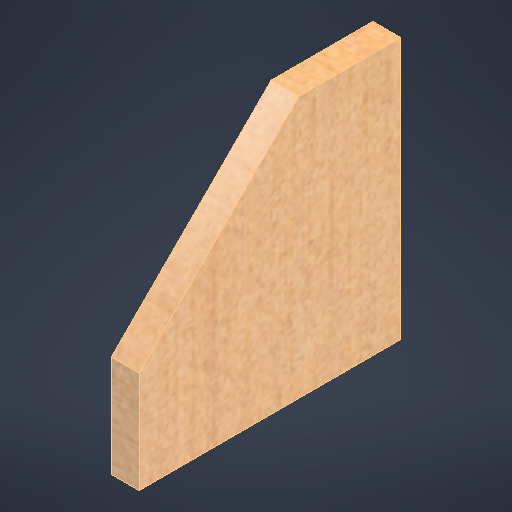
# Autodesk Inventor part: turret_lift
Saved by Autodesk Inventor 2026.2 (Build 302298000, 298)
## iProperties
Created: 2026-01-17
Part Number: turret_lift
Material: Pine
Document SubType Name: Modeling
Designer: User
Density: 0.570257 g/cm^3
Appearance: Yellow Pine - Solid Natural Low Gloss
Author: User
Autodesk Inventor part; units mm, degrees
ref_plane "YZ Plane" through (0, 0, 0) normal (1, 0, 0) x (0, 1, 0)
ref_plane "XZ Plane" through (0, 0, 0) normal (0, 1, 0) x (-1, 0, 0)
ref_plane "XY Plane" through (0, 0, 0) normal (0, 0, 1) x (1, 0, 0)
sketch "Sketch1" plane through (0, 0, 0) normal (1, 0, 0) x (0, 1, 0)
  line L0 (0, 0) -> (90, 0)
  line L1 (90, 0) -> (90, 35)
  line L2 (90, 35) -> (0, 35)
  line L3 (0, 35) -> (0, 0)
  line L4 (90, 35) -> (35, 90)
  line L5 (90, 35) -> (217.2792, 35) construction
  line L6 (0, 90) -> (0, 35)
  line L7 (0, 90) -> (35, 90)
  dimension "d0" = 90
  dimension "d1" = 35
  dimension "d2" = 135
  dimension "d6" = 90
  constraints: 16 end point, 2 horizontal, 2 parallel, 2 perpendicular, 1 vertical
  measures "d0" distance of L0.start L0.end
  measures "d1" distance of L0.end L1.end
  measures "d2" angle of L5 L4
  measures "d6" distance between parallel lines of L0 L7
extrude "Extrusion1" add sketch "Sketch1" along normal blind 9.5813
equation "\"d6\" = d0"
body "Solid1"
